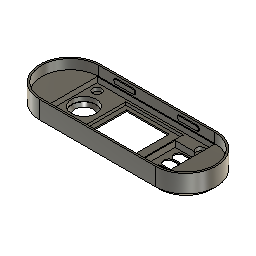
OP_Upper (Autodesk Fusion 360 design; units mm, degrees)
Autodesk Fusion 360 part; units mm, degrees
note: some values were not read from the file. Chosen so that the rebuilt part matches the saved one: which face or edge a step refers to; a side. Set by a fixed rule: which sketch regions a step uses.
sketch "Sketch1" plane through (0, 0, 0) normal (0, 0, 1) x (1, 0, 0)
  arc A0 (32.75, -17.25) -> (32.75, 17.25) centre (32.75, 0) ccw
  line L0 (32.75, -17.25) -> (-32.75, -17.25)
  line L1 (-32.75, 17.25) -> (32.75, 17.25)
  arc A1 (-32.75, 17.25) -> (-32.75, -17.25) centre (-32.75, 0) ccw
extrude "Extrude1" add sketch "Sketch1" along normal blind 9
sketch "Sketch2" plane through (0, 0, 9) normal (0, 0, 1) x (-1, 0, 0)
  arc A0 (-32.75, 17.25) -> (-32.75, -17.25) centre (-32.75, 0) ccw
  line L0 (-32.75, -17.25) -> (32.75, -17.25)
  arc A1 (32.75, -17.25) -> (32.75, 17.25) centre (32.75, 0) ccw
  line L1 (32.75, 17.25) -> (-32.75, 17.25)
  line L2 (32.75, 15.25) -> (-32.75, 15.25)
  arc A2 (-32.75, 15.25) -> (-32.75, -15.25) centre (-32.75, 0) ccw
  line L3 (-32.75, -15.25) -> (32.75, -15.25)
  arc A3 (32.75, -15.25) -> (32.75, 15.25) centre (32.75, 0) ccw
  dimension "d3" = -2
extrude "Extrude2" cut sketch "Sketch2" against normal blind 8 contours L2 A2 L3 A3
sketch "Sketch3" plane through (0, 0, 9) normal (0, 0, 1) x (-1, 0, 0)
  line L0 (-32.75, 15.25) -> (32.75, 15.25)
  arc A0 (32.75, -15.25) -> (32.75, 15.25) centre (32.75, 0) ccw
  line L1 (32.75, -15.25) -> (-32.75, -15.25)
  arc A1 (-32.75, 15.25) -> (-32.75, -15.25) centre (-32.75, 0) ccw
  arc A2 (-32.75, 17.25) -> (-32.75, -17.25) centre (-32.75, 0) ccw
  line L2 (-32.75, -17.25) -> (32.75, -17.25)
  arc A3 (32.75, -17.25) -> (32.75, 17.25) centre (32.75, 0) ccw
  line L3 (32.75, 17.25) -> (-32.75, 17.25)
  line L4 (32.75, 16.25) -> (-32.75, 16.25)
  arc A4 (-32.75, 16.25) -> (-32.75, -16.25) centre (-32.75, 0) ccw
  line L5 (-32.75, -16.25) -> (32.75, -16.25)
  arc A5 (32.75, -16.25) -> (32.75, 16.25) centre (32.75, 0) ccw
  dimension "d6" = -1
extrude "Extrude3" cut sketch "Sketch3" against normal blind 2 contours L4 A4 L5 A5
sketch "Sketch4" plane through (0, 0, 1) normal (0, 0, 1) x (-1, 0, 0)
  arc A0 (32.75, -15.25) -> (32.75, 15.25) centre (32.75, 0) ccw
  line L0 (32.75, 15.25) -> (-32.75, 15.25)
  arc A1 (-32.75, 15.25) -> (-32.75, -15.25) centre (-32.75, 0) ccw
  line L1 (-32.75, -15.25) -> (32.75, -15.25)
  line L2 (15.75, 14) -> (15.75, -14.5)
  line L3 (-16.75, 14) -> (15.75, 14)
  line L4 (15.75, -14.5) -> (-16.75, -14.5)
  line L5 (-16.75, -14.5) -> (-16.75, 14)
  line L6 (-28.25, 8.5) -> (-21.25, 8.5)
  line L7 (-21.25, 8.5) -> (-21.25, -8.5)
  line L8 (-21.25, -8.5) -> (-28.25, -8.5)
  line L9 (-28.25, -8.5) -> (-28.25, 8.5)
  circle A2 centre (29.25, -11.75) radius 1.5
  circle A3 centre (29.25, 11.75) radius 1.5
  circle A4 centre (-29.25, -11.75) radius 1.5
  circle A5 centre (-29.25, 11.75) radius 1.5
  dimension "d27" = 3
  dimension "d28" = 3
  dimension "d29" = 3
  dimension "d30" = 3
  measures "d27" diameter of A2
  measures "d28" diameter of A3
  measures "d29" diameter of A4
  measures "d30" diameter of A5
extrude "Extrude4" cut sketch "Sketch4" against normal blind 1 contours L2 L3 L4 L5 | L6 L7 L8 L9
extrude "Extrude5" add 1 faces at (10.9167, -16.9167, 9) along direction (0, 0, 1) blind 1
extrude "Extrude6" add 1 faces at (-10.9167, -15.9167, 7) along direction (0, 0, 1) blind 1
extrude "Extrude9" add 1 faces at (28.25, 2.8333, 0.6667) along direction (-1, 0, 0) blind 0.5
extrude "Extrude10" add 1 faces at (-27.0833, -4.6667, 1) along direction (0, 0, 1) blind 1
extrude "Extrude11" add 1 faces at (-27.0833, -4.6667, 0) along direction (0, 0, -1) blind 1
sketch "Sketch5" plane through (0, 0, -1) normal (0, 0, -1) x (1, 0, 0)
  line L0 (-15.75, -14.5) -> (-15.75, 14)
  line L1 (-15.75, 14) -> (16.75, 14)
  line L2 (16.75, 14) -> (16.75, -14.5)
  line L3 (16.75, -14.5) -> (-15.75, -14.5)
  line L4 (21.25, -8.5) -> (21.25, 8.5)
  line L5 (21.25, 8.5) -> (27.75, 8.5)
  line L6 (27.75, 8.5) -> (27.75, -8.5)
  line L7 (27.75, -8.5) -> (21.25, -8.5)
  arc A0 (32.75, -17.25) -> (32.75, 17.25) centre (32.75, 0) ccw
  line L8 (32.75, 17.25) -> (-32.75, 17.25)
  arc A1 (-32.75, 17.25) -> (-32.75, -17.25) centre (-32.75, 0) ccw
  line L9 (-32.75, -17.25) -> (32.75, -17.25)
  circle A2 centre (29.25, -11.75) radius 2.5
  circle A3 centre (29.25, 11.75) radius 2.5
  circle A4 centre (-29.25, 11.75) radius 2.5
  circle A5 centre (-29.25, -11.75) radius 2.5
  dimension "d35" = 5
  dimension "d36" = 5
  dimension "d37" = 5
  dimension "d38" = 5
  measures "d35" diameter of A2
  measures "d36" diameter of A3
  measures "d37" diameter of A4
  measures "d38" diameter of A5
extrude "Extrude14" cut 1 faces at (-27.0833, -4.6667, 2) along direction (0, 0, -1) blind 0.5
sketch "Sketch6" plane through (-15.75, 0, 0) normal (1, 0, 0) x (0, 1, 0)
  line L0 (14.5, 1.5) -> (-14, 1.5)
  line L1 (-14, 1.5) -> (-14, -1)
  line L2 (-14, -1) -> (14.5, -1)
  line L3 (14.5, -1) -> (14.5, 1.5)
  line L4 (-0.0213, -1) -> (-0.0213, -0.2) construction
  line L5 (-0.0213, -0.2) -> (14.5, -0.2)
  line L6 (-0.0213, -0.2) -> (-14, -0.2)
  dimension "d57" = 0.8
  constraint coincident L2 L4.start
  constraint perpendicular L2 L4
  constraint coincident L3 L5.end
  constraint perpendicular L3 L5
  constraint coincident L1 L6.end
  constraint perpendicular L1 L6
  measures "d57" distance of L4.start L4.end
extrude "Extrude19" add sketch "Sketch6" along normal blind 2.5 contours L1 L2 L3 L5 L6
sketch "Sketch7" plane through (0, -14, 0) normal (0, 1, 0) x (-1, 0, 0)
  line L0 (13.25, -0.2) -> (15.75, -0.2)
  line L1 (15.75, -0.2) -> (15.75, 1.5)
  line L2 (15.75, 1.5) -> (-16.75, 1.5)
  line L3 (-16.75, 1.5) -> (-16.75, -1)
  line L4 (-16.75, -1) -> (13.25, -1)
  line L5 (13.25, -1) -> (13.25, -0.2)
  line L6 (13.25, -0.2) -> (-16.75, -0.2)
  constraint coincident L0.start L5.end
  constraint coincident L3 L6.end
  constraint perpendicular L3 L6
extrude "Extrude20" add sketch "Sketch7" along normal blind 2 contours L3 L4 L5 L6
sketch "Sketch8" plane through (16.75, 0, 0) normal (-1, 0, 0) x (0, -1, 0)
  line L0 (12, -0.2) -> (14, -0.2)
  line L1 (14, -0.2) -> (14, 1.5)
  line L2 (14, 1.5) -> (-14.5, 1.5)
  line L3 (-14.5, 1.5) -> (-14.5, -1)
  line L4 (-14.5, -1) -> (12, -1)
  line L5 (12, -1) -> (12, -0.2)
  line L6 (12, -0.2) -> (-14.5, -0.2)
  constraint coincident L0.start L5.end
  constraint coincident L3 L6.end
  constraint perpendicular L3 L6
extrude "Extrude21" add sketch "Sketch8" along normal blind 6 contours L3 L4 L5 L6
sketch "Sketch9" plane through (0, 14.5, 0) normal (0, -1, 0) x (1, 0, 0)
  line L0 (10.75, -0.2) -> (16.75, -0.2)
  line L1 (16.75, -0.2) -> (16.75, 1.5)
  line L2 (16.75, 1.5) -> (-15.75, 1.5)
  line L3 (-15.75, 1.5) -> (-15.75, -0.2)
  line L4 (-15.75, -0.2) -> (-13.25, -0.2)
  line L5 (-13.25, -0.2) -> (-13.25, -1)
  line L6 (-13.25, -1) -> (10.75, -1)
  line L7 (10.75, -1) -> (10.75, -0.2)
  line L8 (10.75, -0.2) -> (-13.25, -0.2)
  constraint coincident L0.start L7.end
  constraint coincident L4.end L5.start
extrude "Extrude22" add sketch "Sketch9" along normal blind 2 contours L5 L6 L7 L8
sketch "Sketch10" plane through (0, 0, -1) normal (0, 0, -1) x (1, 0, 0)
  line L0 (21.25, 8.5) -> (27.75, 8.5)
  line L1 (27.75, -8.5) -> (21.25, -8.5)
  line L2 (-26.0471, -6.3671) -> (-24.6329, -6.3671) construction
  line L3 (-25.34, -5.66) -> (-25.34, -7.0742) construction
  line L4 (21.25, -8.5) -> (21.25, 8.5)
  line L5 (27.75, 8.5) -> (27.75, -8.5)
  arc A0 (32.75, -17.25) -> (32.75, 17.25) centre (32.75, 0) ccw
  line L6 (32.75, 17.25) -> (-32.75, 17.25)
  arc A1 (-32.75, 17.25) -> (-32.75, -17.25) centre (-32.75, 0) ccw
  line L7 (-32.75, -17.25) -> (32.75, -17.25)
  line L8 (10.75, -12.5) -> (-13.25, -12.5)
  line L9 (-13.25, -12.5) -> (-13.25, 12)
  line L10 (-13.25, 12) -> (10.75, 12)
  line L11 (10.75, 12) -> (10.75, -12.5)
extrude "Extrude24" cut 1 faces at (21.25, -2.8333, 0.6667) along direction (-1, 0, 0) blind 1
extrude "Extrude25" cut 1 faces at (27.75, 2.8333, 0.6667) along direction (1, 0, 0) blind 1
extrude "Extrude26" add 1 faces at (-26.25, -4, -1) along direction (0, 0, -1) blind 0.5
sketch "Sketch11" plane through (0, 0, 1.5) normal (0, 0, 1) x (-1, 0, 0)
  line L0 (15.75, 14) -> (15.75, -14.5)
  line L1 (15.75, -14.5) -> (-16.75, -14.5)
  line L2 (-16.75, -14.5) -> (-16.75, 14)
  line L3 (-16.75, 14) -> (15.75, 14)
  line L4 (-20.25, -8.5) -> (-28.75, -8.5)
  line L5 (-28.75, -8.5) -> (-28.75, 8.5)
  line L6 (-28.75, 8.5) -> (-20.25, 8.5)
  line L7 (-20.25, 8.5) -> (-20.25, -8.5)
  arc A0 (32.75, -15.25) -> (32.75, 15.25) centre (32.75, 0) ccw
  line L8 (32.75, 15.25) -> (-32.75, 15.25)
  arc A1 (-32.75, 15.25) -> (-32.75, -15.25) centre (-32.75, 0) ccw
  line L9 (-32.75, -15.25) -> (32.75, -15.25)
  line L10 (-28.75, -8.5) -> (-31.75, -8.5)
  line L11 (-28.75, 8.5) -> (-31.75, 8.5)
  line L12 (-31.75, 8.5) -> (-31.75, -8.5)
  line L13 (-20.25, -8.5) -> (-17.25, -8.5)
  line L14 (-20.25, 8.5) -> (-17.25, 8.5)
  line L15 (-17.25, -8.5) -> (-17.25, 8.5)
  dimension "d82" = 3
  dimension "d83" = 3
  dimension "d84" = 3
  dimension "d85" = 3
  constraint coincident L4.end L5.start
  constraint perpendicular L5 L10
  constraint coincident L5.end L6.start
  constraint perpendicular L5 L11
  constraint coincident L4.start L7.end
  constraint perpendicular L7 L13
  constraint coincident L6.end L7.start
  constraint perpendicular L7 L14
  measures "d82" distance of L4.end L10.end
  measures "d83" distance of L5.end L11.end
  measures "d84" distance of L4.start L13.end
  measures "d85" distance of L6.end L14.end
extrude "Extrude27" cut sketch "Sketch11" against normal blind 2.6 contours L7 L13 L14 L15 | L5 L10 L11 L12
sketch "Sketch12" plane through (0, 0, 1.5) normal (0, 0, 1) x (-1, 0, 0)
  arc A0 (32.75, -15.25) -> (32.75, 15.25) centre (32.75, 0) ccw
  line L0 (32.75, 15.25) -> (-32.75, 15.25)
  arc A1 (-32.75, 15.25) -> (-32.75, -15.25) centre (-32.75, 0) ccw
  line L1 (-32.75, -15.25) -> (32.75, -15.25)
  line L2 (15.75, 14) -> (15.75, -14.5)
  line L3 (15.75, -14.5) -> (-16.75, -14.5)
  line L4 (-16.75, -14.5) -> (-16.75, 14)
  line L5 (-16.75, 14) -> (15.75, 14)
  line L6 (-31.75, 8.5) -> (-17.25, 8.5)
  line L7 (-17.25, 8.5) -> (-17.25, -8.5)
  line L8 (-17.25, -8.5) -> (-31.75, -8.5)
  line L9 (-31.75, -8.5) -> (-31.75, 8.5)
sketch "Sketch13" plane through (0, 0, 1.5) normal (0, 0, 1) x (-1, 0, 0)
  arc A0 (32.75, -15.25) -> (32.75, 15.25) centre (32.75, 0) ccw
  line L0 (32.75, 15.25) -> (-32.75, 15.25)
  arc A1 (-32.75, 15.25) -> (-32.75, -15.25) centre (-32.75, 0) ccw
  line L1 (-32.75, -15.25) -> (32.75, -15.25)
  line L2 (15.75, 14) -> (15.75, -14.5)
  line L3 (15.75, -14.5) -> (-16.75, -14.5)
  line L4 (-16.75, -14.5) -> (-16.75, 14)
  line L5 (-16.75, 14) -> (15.75, 14)
  line L6 (-31.75, 8.5) -> (-17.25, 8.5)
  line L7 (-17.25, 8.5) -> (-17.25, -8.5)
  line L8 (-17.25, -8.5) -> (-31.75, -8.5)
  line L9 (-31.75, -8.5) -> (-31.75, 8.5)
  circle A2 centre (25.34, -0.3536) radius 5.25
  circle A3 centre (25.34, -0.3536) radius 7
  dimension "d102" = 10.5
  dimension "d105" = 14
  constraint concentric A2 A3
  measures "d102" diameter of A2
  measures "d105" diameter of A3
extrude "Extrude32" cut sketch "Sketch13" against normal up to surface (3 mm away) contours A2
extrude "Extrude34" add 1 faces at (35.8173, 0.4297, -1.5) along direction (0, 0, -1) blind 1
extrude "Extrude35" cut sketch "Sketch13" against normal blind 2.5 contours A3
chamfer "Chamfer14" distance 1.5 angle 45 1 edges at (-20.4453, 2.252, -1)
chamfer "Chamfer16" distance 1.5 angle 45 4 edges at (-1.25, -12, -2.5) (-13.25, 0.25, -2.5) (-1.25, 12.5, -2.5) (10.75, 0.25, -2.5)
sketch "Sketch14" plane through (0, 0, -1.1) normal (0, 0, 1) x (-1, 0, 0)
  line L0 (-20.25, 8.5) -> (-20.25, -8.5)
  line L1 (-20.25, -8.5) -> (-17.25, -8.5)
  line L2 (-17.25, -8.5) -> (-17.25, 8.5)
  line L3 (-17.25, 8.5) -> (-20.25, 8.5)
  line L4 (-28.75, 8.5) -> (-28.75, -8.5) construction
  line L5 (-28.75, 0) -> (-28.75, -2.6) construction
  line L6 (-17.25, -8.5) -> (-31.75, -8.5) construction
  line L7 (-28.75, -8.5) -> (-28.75, -3.3) construction
  line L8 (-28.75, 0) -> (-28.75, 2.6) construction
  line L9 (-28.75, 8.5) -> (-28.75, 3.3) construction
  line L10 (-28.75, -3.3) -> (-20.25, -3.3) construction
  line L11 (-28.75, -2.6) -> (-20.25, -2.6) construction
  line L12 (-28.75, 2.6) -> (-20.25, 2.6) construction
  line L13 (-28.75, 3.3) -> (-20.25, 3.3) construction
  line L14 (-28.75, -8.5) -> (-27, -8.5)
  line L15 (-28.75, -3.3) -> (-27, -3.3)
  line L16 (-20.25, -8.5) -> (-22, -8.5)
  line L17 (-20.25, -3.3) -> (-22, -3.3)
  line L18 (-28.75, -2.6) -> (-27, -2.6)
  line L19 (-20.25, -2.6) -> (-22, -2.6)
  line L20 (-28.75, 3.3) -> (-27, 3.3)
  line L21 (-20.25, 3.3) -> (-22, 3.3)
  arc A0 (-27, -3.3) -> (-27, -8.5) centre (-25.9436, -5.9) ccw
  arc A1 (-22, -8.5) -> (-22, -3.3) centre (-23.0564, -5.9) ccw
  arc A2 (-27, 2.6) -> (-27, -2.6) centre (-25.9436, 0) ccw
  arc A3 (-27, 8.5) -> (-27, 3.3) centre (-25.9436, 5.9) ccw
  arc A4 (-22, -2.6) -> (-22, 2.6) centre (-23.0564, 0) ccw
  arc A5 (-22, 3.3) -> (-22, 8.5) centre (-23.0564, 5.9) ccw
  line L22 (-22, -3.3) -> (-27, -3.3)
  line L23 (-22, -2.6) -> (-27, -2.6)
  line L24 (-22, 2.6) -> (-27, 2.6)
  line L25 (-22, 3.3) -> (-27, 3.3)
  line L26 (-28.75, -8.5) -> (-28.75, 8.5)
  line L27 (-28.75, 8.5) -> (-27, 8.5)
  line L28 (-22, 8.5) -> (-20.25, 8.5)
  dimension "d123" = 2.6
  dimension "d124" = 5.2
  dimension "d125" = 2.6
  dimension "d126" = 5.2
  dimension "d127" = 1.75
  dimension "d128" = 1.75
  dimension "d129" = 1.75
  dimension "d130" = 1.75
  dimension "d131" = 1.75
  dimension "d132" = 1.75
  dimension "d133" = 1.75
  dimension "d134" = 1.75
  constraint midpoint L4 L5.start
  constraint parallel L4 L5
  constraint coincident L4.end L7.start
  constraint perpendicular L6 L7
  constraint parallel L4 L8
  constraint coincident L4.start L9.start
  constraint parallel L4 L9
  constraint coincident L0 L10.end
  constraint perpendicular L0 L10
  constraint coincident L0 L11.end
  constraint perpendicular L0 L11
  constraint coincident L0 L12.end
  constraint perpendicular L0 L12
  constraint coincident L0 L13.end
  constraint perpendicular L0 L13
  constraint perpendicular L4 L14
  constraint perpendicular L4 L15
  constraint coincident L0.end L1.start
  constraint perpendicular L0 L16
  constraint perpendicular L0 L17
  constraint perpendicular L4 L18
  constraint perpendicular L0 L19
  constraint perpendicular L4 L20
  constraint perpendicular L0 L21
  constraint tangent L4 A0
  constraint parallel L12 L24
  constraint perpendicular L4 L27
  constraint coincident L0.start L3.end
  constraint perpendicular L0 L28
  measures "d123" distance of L5.start L5.end
  measures "d124" distance of L4.end L7.end
  measures "d125" distance of L5.start L8.end
  measures "d126" distance of L4.start L9.end
  measures "d127" distance of L4.end L14.end
  measures "d128" distance of L7.end L15.end
  measures "d129" distance of L0.end L16.end
  measures "d130" distance of L10.end L17.end
  measures "d131" distance of L5.end L18.end
  measures "d132" distance of L11.end L19.end
  measures "d133" distance of L9.end L20.end
  measures "d134" distance of L13.end L21.end
extrude "Extrude36" add sketch "Sketch14" against normal up to surface (1.4 mm away) contours L0 L19 A4 | L0 L15 L17 L18 L19 L22 L23 L26 | L0 L17 A1 | L0 L20 L21 A2 A4 L24 L25 L26 | L0 L16 A1 | L14 A0 L26 | A3 L26 L27 | L0 L21 A5 | L18 A2 L26 | L15 A0 L26 | L0 A5 L28 | L20 A3 L26
extrude "Extrude37" cut 1 faces at (18.25, 0, -1.1) along direction (0, 0, -1) blind 0.4
extrude "Extrude38" cut 1 faces at (-10.9167, -15.9167, 8) along direction (0, 0, -1) blind 2
sketch "Sketch17" plane through (0, 0, 1.5) normal (0, 0, 1) x (-1, 0, 0)
  circle A0 centre (25.34, -0.3536) radius 7
  arc A1 (32.75, -15.25) -> (32.75, 15.25) centre (32.75, 0) ccw
  line L0 (32.75, 15.25) -> (-32.75, 15.25)
  arc A2 (-32.75, 15.25) -> (-32.75, -15.25) centre (-32.75, 0) ccw
  line L1 (-32.75, -15.25) -> (32.75, -15.25)
  line L2 (15.75, 14) -> (15.75, -14.5)
  line L3 (15.75, -14.5) -> (-16.75, -14.5)
  line L4 (-16.75, -14.5) -> (-16.75, 14)
  line L5 (-16.75, 14) -> (15.75, 14)
  line L6 (-31.75, 8.5) -> (-17.25, 8.5)
  line L7 (-17.25, 8.5) -> (-17.25, -8.5)
  line L8 (-17.25, -8.5) -> (-31.75, -8.5)
  line L9 (-31.75, -8.5) -> (-31.75, 8.5)
  line L10 (29.5, -15.25) -> (25.75, -15.25)
  arc A3 (29.5, -15.25) -> (32.75, -12) centre (29.5, -12) ccw
  line L11 (32.75, 12) -> (32.75, -12)
  arc A4 (32.75, 12) -> (29.5, 15.25) centre (29.5, 12) ccw
  line L12 (-29.5, 15.25) -> (29.5, 15.25)
  arc A5 (-29.5, 15.25) -> (-32.75, 12) centre (-29.5, 12) ccw
  line L13 (-32.75, -12) -> (-32.75, 12)
  arc A6 (-32.75, -12) -> (-29.5, -15.25) centre (-29.5, -12) ccw
  line L14 (-26.35, -15.25) -> (-29.5, -15.25)
  line L15 (25.75, -15.25) -> (-26.35, -15.25)
  line L16 (32.95, 12) -> (32.95, -12)
  arc A7 (29.5, -15.45) -> (32.95, -12) centre (29.5, -12) ccw
  line L17 (29.5, -15.45) -> (25.75, -15.45)
  line L18 (25.75, -15.45) -> (-26.35, -15.45)
  line L19 (-26.35, -15.45) -> (-29.5, -15.45)
  arc A8 (-32.95, -12) -> (-29.5, -15.45) centre (-29.5, -12) ccw
  line L20 (-32.95, -12) -> (-32.95, 12)
  arc A9 (-29.5, 15.45) -> (-32.95, 12) centre (-29.5, 12) ccw
  line L21 (-29.5, 15.45) -> (29.5, 15.45)
  arc A10 (32.95, 12) -> (29.5, 15.45) centre (29.5, 12) ccw
  line L22 (29.5, 15.25) -> (29.5, 15.45)
  line L23 (29.5, -15.25) -> (29.5, -15.45)
  line L24 (-29.5, -15.25) -> (-29.5, -15.45)
  line L25 (-29.5, 15.25) -> (-29.5, 15.45)
  dimension "d152" = 0.2
  constraint parallel L1 L15
  constraint vertical L22
  constraint vertical L23
  constraint coincident L17 A7.start
  constraint coincident A7 L17.start
  constraint vertical L24
  constraint coincident A8 L19.end
  constraint coincident L19 A8.end
extrude "Extrude42" cut sketch "Sketch17" along normal up to surface (4.5 mm away) contours L1 A7 L23 | L0 A10 L22 | L1 L10 L14 L15 L17 L18 L19 L23 L24 | L0 L12 L21 L22 L25 | L0 A9 L25 | L1 A8 L24
extrude "Extrude43" add sketch "Sketch17" along normal blind 3 contours A1 L0 L1 L16 A7 A10 | L0 A2 L1 A8 L20 A9
extrude "Extrude44" cut 1 faces at (42.3491, 12.6462, 6) along direction (0, 0, -1) blind 1
extrude "Extrude45" cut 1 faces at (10.9167, -16.9167, 10) along direction (0, 0, -1) blind 1
sketch "Sketch18" plane through (0, 16.25, 0) normal (0, -1, 0) x (1, 0, 0)
  line L0 (32.75, 9) -> (-32.75, 9)
  line L1 (-32.75, 9) -> (-32.75, 5)
  line L2 (-32.75, 5) -> (32.75, 5)
  line L3 (32.75, 5) -> (32.75, 9)
  line L4 (-32.75, 7) -> (-22.75, 7) construction
  line L5 (32.75, 7) -> (22.75, 7) construction
  line L6 (-22.75, 8.5) -> (-13.25, 8.5)
  line L7 (-13.25, 5.5) -> (-22.75, 5.5)
  arc A0 (-22.75, 8.5) -> (-22.75, 5.5) centre (-22.75, 7) ccw
  arc A1 (-13.25, 5.5) -> (-13.25, 8.5) centre (-13.25, 7) ccw
  line L8 (13.25, 8.5) -> (22.75, 8.5)
  arc A2 (13.25, 8.5) -> (13.25, 5.5) centre (13.25, 7) ccw
  line L9 (22.75, 5.5) -> (13.25, 5.5)
  arc A3 (22.75, 5.5) -> (22.75, 8.5) centre (22.75, 7) ccw
  dimension "d161" = 10
  dimension "d162" = 10
  constraint midpoint L1 L4.start
  constraint perpendicular L1 L4
  constraint midpoint L3 L5.start
  constraint perpendicular L3 L5
  measures "d161" distance of L4.start L4.end
  measures "d162" distance of L5.start L5.end
extrude "Extrude46" add sketch "Sketch18" along normal blind 0.3 contours L6 L7 A0 A1 | L8 A2 L9 A3
chamfer "Chamfer19" distance 0.3 angle 45 8 edges at (-18, 15.95, 8.5) (-24.25, 15.95, 7) (-18, 15.95, 5.5) (-11.75, 15.95, 7) (18, 15.95, 8.5) (11.75, 15.95, 7) (18, 15.95, 5.5) (24.25, 15.95, 7)
sketch "Sketch19" plane through (0, -16.25, 0) normal (0, 1, 0) x (-1, 0, 0)
  line L0 (32.75, 9) -> (-32.75, 9)
  line L1 (-32.75, 9) -> (-32.75, 5)
  line L2 (-32.75, 5) -> (32.75, 5)
  line L3 (32.75, 5) -> (32.75, 9)
  line L4 (-32.75, 7) -> (-9.35, 7) construction
  line L5 (-9.35, 8.5) -> (0.15, 8.5)
  arc A0 (-9.35, 8.5) -> (-9.35, 5.5) centre (-9.35, 7) ccw
  line L6 (0.15, 5.5) -> (-9.35, 5.5)
  arc A1 (0.15, 5.5) -> (0.15, 8.5) centre (0.15, 7) ccw
  dimension "d166" = 23.4
  constraint midpoint L1 L4.start
  constraint perpendicular L1 L4
  measures "d166" distance of L4.start L4.end
extrude "Extrude47" add sketch "Sketch19" along normal blind 0.3 contours L5 A0 L6 A1
chamfer "Chamfer20" distance 0.3 angle 45 4 edges at (4.6, -15.95, 8.5) (10.85, -15.95, 7) (4.6, -15.95, 5.5) (-1.65, -15.95, 7)
chamfer "Chamfer21" distance 2.4 angle 45 4 edges at (0, -17.25, -2.5) (-50, 0, -2.5) (0, 17.25, -2.5) (50, 0, -2.5) measured on face at (10.9167, -17.25, 1.3333) measured on face at (-45.6837, -11.4141, 5.1667) measured on face at (-10.9167, 17.25, 1.3333) measured on face at (48.4735, 7.0947, 5.1667)
sketch "Sketch20" plane through (0, 8.5, 0) normal (0, -1, 0) x (1, 0, 0)
  line L0 (22, -1.5) -> (22, -2.5)
  line L1 (22, -2.5) -> (27, -2.5)
  line L2 (27, -2.5) -> (27, -1.5)
  line L3 (27, -1.5) -> (31.75, -1.5)
  line L4 (31.75, -1.5) -> (31.75, 1.5)
  line L5 (31.75, 1.5) -> (17.25, 1.5)
  line L6 (17.25, 1.5) -> (17.25, -1.5)
  line L7 (17.25, -1.5) -> (22, -1.5)
  line L8 (22, -1.5) -> (27, -1.5)
  constraint coincident L0.start L7.end
  constraint coincident L2.end L3.start
extrude "Extrude48" cut sketch "Sketch20" against normal blind 1 contours L3 L4 L5 L6 L7 L8
sketch "Sketch21" plane through (0, -8.5, 0) normal (0, 1, 0) x (-1, 0, 0)
  line L0 (-17.25, -1.5) -> (-17.25, 1.5)
  line L1 (-17.25, 1.5) -> (-31.75, 1.5)
  line L2 (-31.75, 1.5) -> (-31.75, -1.5)
  line L3 (-31.75, -1.5) -> (-27, -1.5)
  line L4 (-27, -1.5) -> (-27, -2.5)
  line L5 (-27, -2.5) -> (-22, -2.5)
  line L6 (-22, -2.5) -> (-22, -1.5)
  line L7 (-22, -1.5) -> (-17.25, -1.5)
  line L8 (-27, -1.5) -> (-22, -1.5)
  constraint coincident L3.end L4.start
  constraint coincident L6.end L7.start
extrude "Extrude49" cut sketch "Sketch21" against normal blind 1 contours L0 L1 L2 L3 L7 L8
sketch "Sketch22" plane through (0, 0, 1.5) normal (0, 0, 1) x (-1, 0, 0)
  arc A0 (-32.95, -12) -> (-29.5, -15.45) centre (-29.5, -12) ccw
  line L0 (-29.5, -15.45) -> (29.5, -15.45)
  arc A1 (29.5, -15.45) -> (32.95, -12) centre (29.5, -12) ccw
  line L1 (32.95, -12) -> (32.95, 12)
  arc A2 (32.95, 12) -> (29.5, 15.45) centre (29.5, 12) ccw
  line L2 (29.5, 15.45) -> (-29.5, 15.45)
  arc A3 (-29.5, 15.45) -> (-32.95, 12) centre (-29.5, 12) ccw
  line L3 (-32.95, 12) -> (-32.95, -12)
  circle A4 centre (25.34, -0.3536) radius 7
  line L4 (15.75, 14) -> (15.75, -14.5)
  line L5 (15.75, -14.5) -> (-16.75, -14.5)
  line L6 (-16.75, -14.5) -> (-16.75, 14)
  line L7 (-16.75, 14) -> (15.75, 14)
  line L8 (-31.75, -9.5) -> (-31.75, 9.5)
  line L9 (-31.75, 9.5) -> (-17.25, 9.5)
  line L10 (-17.25, 9.5) -> (-17.25, -9.5)
  line L11 (-17.25, -9.5) -> (-31.75, -9.5)
  circle A5 centre (-29.25, 11.75) radius 2.5
  circle A6 centre (-29.25, -11.75) radius 2.5
  circle A7 centre (29.25, 11.75) radius 2.5
  circle A8 centre (29.25, -11.75) radius 2.5
extrude "Extrude50" cut sketch "Sketch22" against normal blind 2 contours L11 A6 | L11 A6 | L9 A5 | A7 | A8 picked at (-30.2375, 12.4247)
extrude "Extrude51" cut 1 faces at (42.3491, 12.6462, 5) along direction (0, 0, -1) up to surface (3.5 mm away)
extrude "Extrude52" cut 2 faces at (-37.9525, -0.3799, 4.5) (37.9525, -0.3799, 4.5) along direction (0, 0, 1) up to surface end surface through (0, 0, 1.5) normal (0, 0, 1) offset 0
sketch "Sketch23" plane through (0, 0, 1.5) normal (0, 0, 1) x (-1, 0, 0)
  line L0 (32.75, 16.25) -> (-32.75, 16.25)
  arc A0 (-32.75, 16.25) -> (-32.75, -16.25) centre (-32.75, 0) ccw
  line L1 (-32.75, -16.25) -> (32.75, -16.25)
  arc A1 (32.75, -16.25) -> (32.75, 16.25) centre (32.75, 0) ccw
  arc A2 (-28.1603, 9.5) -> (-30.3397, 9.5) centre (-29.25, 11.75) ccw
  line L2 (-28.1603, 9.5) -> (-17.25, 9.5)
  line L3 (-17.25, 9.5) -> (-17.25, -9.5)
  line L4 (-17.25, -9.5) -> (-28.1603, -9.5)
  arc A3 (-30.3397, -9.5) -> (-28.1603, -9.5) centre (-29.25, -11.75) ccw
  line L5 (-30.3397, -9.5) -> (-31.75, -9.5)
  line L6 (-31.75, -9.5) -> (-31.75, 9.5)
  line L7 (-31.75, 9.5) -> (-30.3397, 9.5)
  line L8 (15.75, 14) -> (15.75, -14.5)
  line L9 (15.75, -14.5) -> (-16.75, -14.5)
  line L10 (-16.75, -14.5) -> (-16.75, 14)
  line L11 (-16.75, 14) -> (15.75, 14)
  circle A4 centre (25.34, -0.3536) radius 7
  circle A5 centre (29.25, -11.75) radius 2.5
  circle A6 centre (29.25, 11.75) radius 2.5
  line L12 (0, -16.25) -> (0, -15.75) construction
  line L13 (0, 16.25) -> (0, 15.75) construction
  line L14 (0, -15.75) -> (-36.75, -15.75)
  line L15 (0, -15.75) -> (36.75, -15.75)
  line L16 (0, 15.75) -> (-36.75, 15.75)
  line L17 (0, 15.75) -> (36.75, 15.75)
  dimension "d186" = 0.5
  dimension "d187" = 0.5
  constraint midpoint L1 L12.start
  constraint vertical L12
  constraint midpoint L0 L13.start
  constraint perpendicular L0 L13
  constraint horizontal L14
  constraint coincident A0 L14.end
  constraint coincident A1 L15.end
  constraint coincident A0 L16.end
  constraint coincident A1 L17.end
  measures "d186" distance of L12.start L12.end
  measures "d187" distance of L13.start L13.end
extrude "Extrude53" add sketch "Sketch23" along normal blind 3 contours L0 A0 A1 L16 L17 | A0 L1 A1 L14 L15
sketch "Sketch24" plane through (0, 0, 1.5) normal (0, 0, 1) x (-1, 0, 0)
  line L0 (-36.75, -15.75) -> (36.75, -15.75)
  arc A0 (36.75, -15.75) -> (36.75, 15.75) centre (32.75, 0) ccw
  line L1 (36.75, 15.75) -> (-36.75, 15.75)
  arc A1 (-36.75, 15.75) -> (-36.75, -15.75) centre (-32.75, 0) ccw
  arc A2 (-28.1603, 9.5) -> (-30.3397, 9.5) centre (-29.25, 11.75) ccw
  line L2 (-28.1603, 9.5) -> (-17.25, 9.5)
  line L3 (-17.25, 9.5) -> (-17.25, -9.5)
  line L4 (-17.25, -9.5) -> (-28.1603, -9.5)
  arc A3 (-30.3397, -9.5) -> (-28.1603, -9.5) centre (-29.25, -11.75) ccw
  line L5 (-30.3397, -9.5) -> (-31.75, -9.5)
  line L6 (-31.75, -9.5) -> (-31.75, 9.5)
  line L7 (-31.75, 9.5) -> (-30.3397, 9.5)
  line L8 (15.75, 14) -> (15.75, -14.5)
  line L9 (15.75, -14.5) -> (-16.75, -14.5)
  line L10 (-16.75, -14.5) -> (-16.75, 14)
  line L11 (-16.75, 14) -> (15.75, 14)
  circle A4 centre (25.34, -0.3536) radius 7
  circle A5 centre (29.25, -11.75) radius 2.5
  circle A6 centre (29.25, 11.75) radius 2.5
  line L12 (32.75, -9) -> (33.25, -9) construction
  line L13 (-32.75, -9) -> (-33.25, -9) construction
  line L14 (33.25, -9) -> (33.25, -15.75)
  line L15 (33.25, -9) -> (33.25, 15.75)
  line L16 (-33.25, -9) -> (-33.25, -15.75)
  line L17 (-33.25, -9) -> (-33.25, 15.75)
  constraint horizontal L12
  constraint horizontal L13
  constraint vertical L14
  constraint coincident L0 L14.end
  constraint coincident L1 L15.end
  constraint perpendicular L1 L15
  constraint coincident L0 L16.end
  constraint perpendicular L0 L16
  constraint coincident L1 L17.end
  constraint perpendicular L1 L17
extrude "Extrude54" add sketch "Sketch24" along normal blind 3 contours L0 L1 A1 L16 L17 | L0 A0 L1 L14 L15
extrude "Extrude55" add 1 faces at (10.9167, -16.9167, 9) along direction (0, 0, 1) blind 1
extrude "Extrude56" cut 1 faces at (18.25, 0, -1.5) along direction (0, 0, -1) blind 0.4
